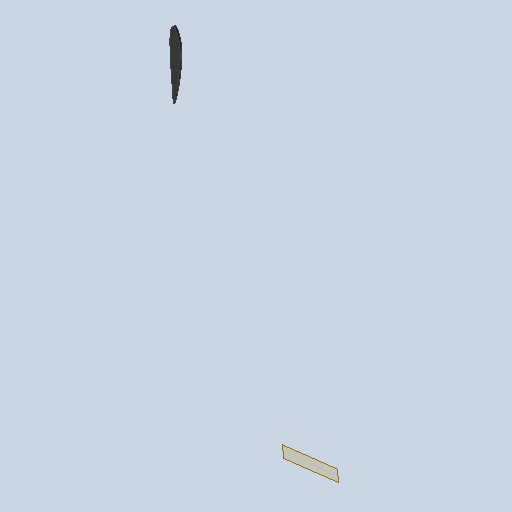
# Autodesk Inventor part: WingCap
Saved by Autodesk Inventor 2025.2 (Build 292293000, 293)
## iProperties
Created: 2025-03-16
Part Number: WingCap
Material: Generic
Document SubType Name: Modeling
Designer: Cupri
Density: 1 g/cm^3
Appearance: Default
Author: Cupri
Autodesk Inventor part; units mm, degrees
ref_plane "YZ Plane" through (0, 0, 0) normal (1, 0, 0) x (0, 1, 0)
ref_plane "XZ Plane" through (0, 0, 0) normal (0, 1, 0) x (-1, 0, 0)
ref_plane "XY Plane" through (0, 0, 0) normal (0, 0, 1) x (1, 0, 0)
ref_plane "Work Plane1" through (463.7305, -1035.5064, 0) normal (0, 0, 1) x (0.1166636, -0.9931715, 0)
sketch "Sketch1" plane through (463.7305, -1035.5064, 0) normal (0, 0, 1) x (0.1166636, -0.9931715, 0)
  line L0 (-1119.3235, -329.4885) -> (-1106.7103, -330.9701) projected
  line L1 (-1106.7103, -330.9701) -> (-1108.1919, -343.5834) projected
  line L2 (-1108.1919, -343.5834) -> (-1120.8052, -342.1018) projected
  line L3 (-1120.8052, -342.1018) -> (-1119.3235, -329.4885) projected
  line L4 (-1023.2686, -358.3554) -> (-1020.9309, -338.4541) projected
  spline S0 degree 4 poles (-1020.9309, -338.4541) (-1026.5338, -336.7537) (-1038.7232, -333.1109) (-1055.1163, -328.7515) (-1079.6641, -323.1903) (-1100.3284, -318.8993) (-1127.386, -315.4589) (-1138.7674, -314.7533) (-1153.2051, -314.4719) (-1164.1562, -314.8378) (-1177.8633, -316.3868) (-1184.0767, -317.949) (-1190.5481, -319.3093) (-1198.4132, -322.9201) (-1200.6065, -324.0146) (-1207.3481, -330.9087) (-1202.2856, -337.2463) (-1200.1655, -338.713) (-1193.1468, -342.4526) (-1187.1056, -344.1727) (-1181.2102, -345.8547) (-1168.0048, -348.531) (-1157.3156, -350.0048) (-1143.0595, -351.6304) (-1131.7178, -352.5935) (-1104.6159, -354.7467) (-1083.3693, -355.9217) (-1058.8468, -356.9821) (-1040.4385, -357.6891) (-1028.9285, -358.141) (-1023.2686, -358.3554) knots 0.096456 0.096456 0.096456 0.096456 0.096456 0.132907 0.173364 0.213741 0.251119 0.285536 0.317038 0.345695 0.372397 0.397199 0.420236 0.440116 0.460308 0.480206 0.498565 0.518053 0.537157 0.556377 0.578869 0.603285 0.629723 0.658222 0.689661 0.724055 0.761412 0.801733 0.842066 0.879452 0.879452 0.879452 0.879452 0.879452 projected
  line L5 (-1020.9309, -338.4541) -> (-1074.8444, -347.7607)
  line L6 (-11.0175, -70.7186) -> (-1195.771, -340.9542)
  line L7 (-959.249, -359.7001) -> (-959.3626, -360.6675) projected
  spline S1 degree 3 poles (-973.6958, -354.1921) (-970.6173, -355.3577) (-968.098, -356.3267) (-962.5104, -358.4635) (-961.9393, -358.6819) (-959.249, -359.7001) knots 0 0 0 0 0.987527 0.987527 1.577405 1.577405 1.577405 1.577405 projected
  spline S2 degree 3 poles (-1020.8864, -338.0757) (-1012.9265, -340.5653) (-1004.9752, -343.1425) (-989.1659, -348.5464) (-980.2142, -351.7501) (-973.6958, -354.1921) knots 0 0 0 0 2.502042 2.502042 5.026236 5.026236 5.026236 5.026236 projected
  ellipse E0 centre (-1001.3774, -340.3673) end of major axis (-1020.8864, -338.0757) minor radius 19.5694 (-1020.8864, -338.0757) -> (-997.2075, -359.4952) ccw projected
  spline S3 degree 3 poles (-959.3626, -360.6675) (-964.8306, -360.5222) (-965.81, -360.5012) (-981.8664, -359.9802) (-989.5369, -359.7357) (-997.2075, -359.4952) knots 0 0 0 0 1.64098 1.64098 3.141934 3.141934 3.141934 3.141934 projected
  line L8 (-1119.3235, -329.4885) -> (-1106.7103, -330.9701) projected
  line L9 (-1106.7103, -330.9701) -> (-1108.1919, -343.5834) projected
  line L10 (-1108.1919, -343.5834) -> (-1120.8052, -342.1018) projected
  line L11 (-1120.8052, -342.1018) -> (-1119.3235, -329.4885) projected
  line L12 (-1023.2686, -358.3554) -> (-1020.9309, -338.4541) projected
  spline S4 degree 4 poles (-1020.9309, -338.4541) (-1026.5338, -336.7537) (-1038.7232, -333.1109) (-1055.1163, -328.7515) (-1079.6641, -323.1903) (-1100.3284, -318.8993) (-1127.386, -315.4589) (-1138.7674, -314.7533) (-1153.2051, -314.4719) (-1164.1562, -314.8378) (-1177.8633, -316.3868) (-1184.0767, -317.949) (-1190.5481, -319.3093) (-1198.4132, -322.9201) (-1200.6065, -324.0146) (-1207.3481, -330.9087) (-1202.2856, -337.2463) (-1200.1655, -338.713) (-1193.1468, -342.4526) (-1187.1056, -344.1727) (-1181.2102, -345.8547) (-1168.0048, -348.531) (-1157.3156, -350.0048) (-1143.0595, -351.6304) (-1131.7178, -352.5935) (-1104.6159, -354.7467) (-1083.3693, -355.9217) (-1058.8468, -356.9821) (-1040.4385, -357.6891) (-1028.9285, -358.141) (-1023.2686, -358.3554) knots 0.096456 0.096456 0.096456 0.096456 0.096456 0.132907 0.173364 0.213741 0.251119 0.285536 0.317038 0.345695 0.372397 0.397199 0.420236 0.440116 0.460308 0.480206 0.498565 0.518053 0.537157 0.556377 0.578869 0.603285 0.629723 0.658222 0.689661 0.724055 0.761412 0.801733 0.842066 0.879452 0.879452 0.879452 0.879452 0.879452 projected
  line L13 (-959.249, -359.7001) -> (-959.3626, -360.6675) projected
  spline S5 degree 3 poles (-973.6958, -354.1921) (-970.6173, -355.3577) (-968.098, -356.3267) (-962.5104, -358.4635) (-961.9393, -358.6819) (-959.249, -359.7001) knots 0 0 0 0 0.987527 0.987527 1.577405 1.577405 1.577405 1.577405 projected
  spline S6 degree 3 poles (-1020.8864, -338.0757) (-1012.9265, -340.5653) (-1004.9752, -343.1425) (-989.1659, -348.5464) (-980.2142, -351.7501) (-973.6958, -354.1921) knots 0 0 0 0 2.502042 2.502042 5.026236 5.026236 5.026236 5.026236 projected
  ellipse E1 centre (-1001.3774, -340.3673) end of major axis (-1020.8864, -338.0757) minor radius 19.5694 (-1020.8864, -338.0757) -> (-997.2075, -359.4952) ccw projected
  spline S7 degree 3 poles (-959.3626, -360.6675) (-964.8306, -360.5222) (-965.81, -360.5012) (-981.8664, -359.9802) (-989.5369, -359.7357) (-997.2075, -359.4952) knots 0 0 0 0 1.64098 1.64098 3.141934 3.141934 3.141934 3.141934 projected
  line L14 (-1020.9309, -338.4541) -> (-1020.8864, -338.0757)
  line L15 (-997.2075, -359.4952) -> (-1023.2686, -358.3554)
  point P0 (-1082.5359, -339.758)
  constraints: 8 end point, 3 other
extrude "Extrusion1" add sketch "Sketch1" along normal blind 6.35 contours S0 L6 L4 | L4 L14 E0 L15 | S0 L6 | E0 S2 S1 L7 S3 L15
sketch "Sketch2" plane through (463.7305, -1035.5064, 0) normal (0, 0, -1) x (-0.1166636, 0.9931715, 0)
  line L0 (1106.7103, -330.9701) -> (1108.1919, -343.5834) projected
  line L1 (1119.3235, -329.4885) -> (1106.7103, -330.9701) projected
  line L2 (1120.8052, -342.1018) -> (1119.3235, -329.4885) projected
  line L3 (1108.1919, -343.5834) -> (1120.8052, -342.1018) projected
  ellipse E0 centre (4.857, -80.0159) end of major axis (4.8635, -79.0121) minor radius 1 projected
  line L4 (1119.3235, -329.4885) -> (1106.7103, -330.9701) projected
  line L5 (1106.7103, -330.9701) -> (1108.1919, -343.5834) projected
  line L6 (1108.1919, -343.5834) -> (1120.8052, -342.1018) projected
  line L7 (1120.8052, -342.1018) -> (1119.3235, -329.4885) projected
  line L8 (959.3626, -360.6675) -> (959.249, -359.7001) projected
  line L9 (1020.8864, -338.0757) -> (1020.9309, -338.4541) projected
  line L10 (1023.2686, -358.3554) -> (997.2075, -359.4952) projected
  point P0 (1082.5359, -339.758)
  constraints: 4 other
extrude "Extrusion2" add sketch "Sketch2" along normal blind 12.7 contours L1 L2 L3 L0
sketch "Sketch3" plane through (463.7305, -1035.5064, 0) normal (0, 0, 1) x (0.1166636, -0.9931715, 0)
  line L0 (-1106.7103, -330.9701) -> (-1108.1919, -343.5834) projected
  line L1 (-1119.3235, -329.4885) -> (-1106.7103, -330.9701) projected
  line L2 (-1120.8052, -342.1018) -> (-1119.3235, -329.4885) projected
  line L3 (-1108.1919, -343.5834) -> (-1120.8052, -342.1018) projected
  point P0 (-1082.5359, -339.758)
extrude "Extrusion3" add sketch "Sketch3" along normal up to surface (6.35 mm away)
body "Solid1"
